Autodesk Fusion 360 part; units mm, degrees
note: some values were not read from the file. Set by a fixed rule: which sketch regions a step uses.
(part 2 of 3)
  line L685 (14.5126, 3.5841) -> (14.4849, 3.5912)
  line L686 (14.4849, 0.409) -> (14.5126, 0.4161)
  line L687 (11.4493, 3.5709) -> (11.4223, 3.5588)
  line L688 (11.209, 0.715) -> (11.2161, 0.6873)
  line L689 (11.5713, 0.4011) -> (11.5999, 0.4001)
  line L690 (14.4568, 0.4039) -> (14.4849, 0.409)
  line L691 (11.3477, 3.5108) -> (11.3254, 3.4913)
  line L692 (14.7988, 0.7713) -> (14.7998, 0.7998)
  line L693 (14.7509, 0.6082) -> (14.7637, 0.6337)
  line L694 (11.2097, 3.2885) -> (11.2043, 3.2594)
  line L695 (14.7022, 0.5379) -> (14.7201, 0.5601)
  line L696 (14.6618, 0.4976) -> (14.6827, 0.517)
  line L697 (14.6827, 0.517) -> (14.7022, 0.5379)
  line L698 (14.5126, 0.4161) -> (14.5397, 0.4251)
  line L699 (14.5916, 0.4488) -> (14.6161, 0.4634)
  line L700 (14.5397, 0.4251) -> (14.566, 0.436)
  line L701 (14.6161, 0.4634) -> (14.6396, 0.4796)
  line L702 (14.7998, 0.7998) -> (14.7998, 3.2004)
  line L703 (14.7836, 0.6872) -> (14.7907, 0.7148)
  line L704 (34.6396, 3.5206) -> (34.6161, 3.5368)
  line L705 (31.4337, 0.4362) -> (31.4601, 0.4253)
  line L706 (31.2634, 0.5838) -> (31.2797, 0.5603)
  line L707 (34.7201, 0.5601) -> (34.7364, 0.5836)
  line L708 (31.4771, 3.581) -> (31.4493, 3.5709)
  line L709 (31.4601, 0.4253) -> (31.4872, 0.4163)
  line L710 (34.3999, 0.3998) -> (34.4284, 0.4009)
  line L711 (31.1999, 3.2001) -> (31.1999, 0.8)
  line L712 (34.6396, 0.4796) -> (34.6618, 0.4976)
  line L713 (31.317, 0.5172) -> (31.3379, 0.4977)
  line L714 (34.7364, 0.5836) -> (34.7509, 0.6082)
  line L715 (31.4082, 0.449) -> (31.4337, 0.4362)
  line L716 (31.564, 3.5987) -> (31.5346, 3.595)
  line L717 (34.6618, 3.5026) -> (34.6396, 3.5206)
  line L718 (34.4284, 3.5993) -> (34.3999, 3.6004)
  line L719 (31.3962, 3.5446) -> (31.3713, 3.5286)
  line L720 (31.3379, 0.4977) -> (31.3602, 0.4798)
  line L721 (34.4284, 0.4009) -> (34.4568, 0.4039)
  line L722 (34.7988, 0.7713) -> (34.7998, 0.7998)
  line L723 (34.5126, 0.4161) -> (34.5397, 0.4251)
  line L724 (31.2097, 3.2885) -> (31.2043, 3.2594)
  line L725 (31.2161, 0.6873) -> (31.2251, 0.6602)
  line L726 (34.4568, 0.4039) -> (34.4849, 0.409)
  line L727 (31.2488, 0.6083) -> (31.2634, 0.5838)
  line L728 (31.1999, 3.2005) -> (31.1999, 3.2001)
  line L729 (31.3836, 0.4635) -> (31.4082, 0.449)
  line L730 (34.4849, 0.409) -> (34.5126, 0.4161)
  line L731 (34.6827, 0.517) -> (34.7022, 0.5379)
  line L732 (31.2009, 0.7715) -> (31.2039, 0.7431)
  line L733 (31.2797, 0.5603) -> (31.2976, 0.5381)
  line L734 (31.209, 0.715) -> (31.2161, 0.6873)
  line L735 (31.2976, 0.5381) -> (31.317, 0.5172)
  line L736 (31.1999, 3.2004) -> (31.1999, 3.2005)
  line L737 (34.3999, 0.4001) -> (34.3999, 0.3998)
  line L738 (34.7637, 0.6337) -> (34.7746, 0.6601)
  line L739 (34.7907, 0.7148) -> (34.7958, 0.7429)
  line L740 (34.7958, 0.7429) -> (34.7988, 0.7713)
  line L741 (34.5916, 0.4488) -> (34.6161, 0.4634)
  line L742 (34.7836, 0.6872) -> (34.7907, 0.7148)
  line L743 (34.5397, 0.4251) -> (34.566, 0.436)
  line L744 (34.6618, 0.4976) -> (34.6827, 0.517)
  line L745 (34.7998, 0.7998) -> (34.7998, 3.2004)
  line L746 (34.7958, 3.2573) -> (34.7907, 3.2854)
  line L747 (34.7836, 3.313) -> (34.7746, 3.3401)
  line L748 (34.6161, 3.5368) -> (34.5916, 3.5514)
  line L749 (31.5346, 3.595) -> (31.5056, 3.5891)
  line L750 (34.3999, 3.6004) -> (34.3999, 3.6002)
  line L751 (31.3046, 3.4702) -> (31.2855, 3.4476)
  line L752 (31.268, 3.4237) -> (31.2524, 3.3985)
  line L753 (34.7201, 3.4401) -> (34.7022, 3.4623)
  line L754 (31.2524, 3.3985) -> (31.2387, 3.3723)
  line L755 (34.7998, 3.2004) -> (34.7988, 3.2289)
  line L756 (31.227, 3.3451) -> (31.2173, 3.3171)
  line L757 (34.5916, 3.5514) -> (34.566, 3.5642)
  line L758 (31.3713, 3.5286) -> (31.3477, 3.5108)
  line L759 (31.4493, 3.5709) -> (31.4223, 3.5588)
  line L760 (34.7988, 3.2289) -> (34.7958, 3.2573)
  line L761 (34.3999, 3.6002) -> (31.5999, 3.6002)
  line L762 (31.4223, 3.5588) -> (31.3962, 3.5446)
  line L763 (34.7637, 3.3665) -> (34.7509, 3.392)
  line L764 (34.7022, 3.4623) -> (34.6827, 3.4832)
  line L765 (31.3254, 3.4913) -> (31.3046, 3.4702)
  line L766 (34.7364, 3.4166) -> (34.7201, 3.4401)
  line L767 (34.7509, 3.392) -> (34.7364, 3.4166)
  line L768 (34.7746, 3.3401) -> (34.7637, 3.3665)
  line L769 (31.5935, 3.6003) -> (31.564, 3.5987)
  line L770 (31.3477, 3.5108) -> (31.3254, 3.4913)
  line L771 (31.2173, 3.3171) -> (31.2097, 3.2885)
  line L772 (34.5126, 3.5841) -> (34.4849, 3.5912)
  line L773 (31.5999, 3.6002) -> (31.5935, 3.6003)
  line L774 (31.5056, 3.5891) -> (31.4771, 3.581)
  line L775 (31.4872, 0.4163) -> (31.5149, 0.4092)
  line L776 (31.2387, 3.3723) -> (31.227, 3.3451)
  line L777 (31.201, 3.2299) -> (31.1999, 3.2004)
  line L778 (34.7907, 3.2854) -> (34.7836, 3.313)
  line L779 (31.1999, 0.8) -> (31.2009, 0.7715)
  line L780 (34.5397, 3.5751) -> (34.5126, 3.5841)
  line L781 (34.566, 3.5642) -> (34.5397, 3.5751)
  line L782 (34.6161, 0.4634) -> (34.6396, 0.4796)
  line L783 (34.6827, 3.4832) -> (34.6618, 3.5026)
  line L784 (31.3602, 0.4798) -> (31.3836, 0.4635)
  line L785 (34.4849, 3.5912) -> (34.4568, 3.5963)
  line L786 (34.4568, 3.5963) -> (34.4284, 3.5993)
  line L787 (31.2855, 3.4476) -> (31.268, 3.4237)
  line L788 (34.566, 0.436) -> (34.5916, 0.4488)
  line L789 (34.7746, 0.6601) -> (34.7836, 0.6872)
  line L790 (31.2039, 0.7431) -> (31.209, 0.715)
  line L791 (31.2043, 3.2594) -> (31.201, 3.2299)
  line L792 (31.2251, 0.6602) -> (31.236, 0.6339)
  line L793 (31.5999, 0.4001) -> (34.3999, 0.4001)
  line L794 (31.5713, 0.4011) -> (31.5999, 0.4001)
  line L795 (31.236, 0.6339) -> (31.2488, 0.6083)
  line L796 (31.5149, 0.4092) -> (31.5429, 0.4041)
  line L797 (34.7022, 0.5379) -> (34.7201, 0.5601)
  line L798 (34.7509, 0.6082) -> (34.7637, 0.6337)
  line L799 (31.5429, 0.4041) -> (31.5713, 0.4011)
  line L800 (51.4223, 3.5588) -> (51.3962, 3.5446)
  line L801 (54.7201, 3.4401) -> (54.7022, 3.4623)
  line L802 (51.3254, 3.4913) -> (51.3046, 3.4702)
  line L803 (51.2855, 3.4476) -> (51.268, 3.4237)
  line L804 (51.2524, 3.3985) -> (51.2387, 3.3723)
  line L805 (54.7637, 0.6337) -> (54.7746, 0.6601)
  line L806 (54.566, 3.5642) -> (54.5397, 3.5751)
  line L807 (51.2797, 0.5603) -> (51.2976, 0.5381)
  line L808 (54.7988, 0.7713) -> (54.7998, 0.7998)
  line L809 (51.317, 0.5172) -> (51.3379, 0.4977)
  line L810 (54.3999, 3.6004) -> (54.3999, 3.6002)
  line L811 (51.3602, 0.4798) -> (51.3836, 0.4635)
  line L812 (54.6161, 0.4634) -> (54.6396, 0.4796)
  line L813 (54.7907, 0.7148) -> (54.7958, 0.7429)
  line L814 (54.7998, 0.7998) -> (54.7998, 3.2004)
  line L815 (54.7022, 3.4623) -> (54.6827, 3.4832)
  line L816 (51.2039, 0.7431) -> (51.209, 0.715)
  line L817 (54.7988, 3.2289) -> (54.7958, 3.2573)
  line L818 (51.5346, 3.595) -> (51.5056, 3.5891)
  line L819 (51.227, 3.3451) -> (51.2173, 3.3171)
  line L820 (54.7022, 0.5379) -> (54.7201, 0.5601)
  line L821 (54.6618, 0.4976) -> (54.6827, 0.517)
  line L822 (54.6396, 3.5206) -> (54.6161, 3.5368)
  line L823 (54.4284, 0.4009) -> (54.4568, 0.4039)
  line L824 (54.7201, 0.5601) -> (54.7364, 0.5836)
  line L825 (54.7509, 0.6082) -> (54.7637, 0.6337)
  line L826 (54.4568, 0.4039) -> (54.4849, 0.409)
  line L827 (51.5999, 0.4001) -> (54.3999, 0.4001)
  line L828 (54.7958, 0.7429) -> (54.7988, 0.7713)
  line L829 (54.5916, 0.4488) -> (54.6161, 0.4634)
  line L830 (51.4601, 0.4253) -> (51.4872, 0.4163)
  line L831 (54.6618, 3.5026) -> (54.6396, 3.5206)
  line L832 (54.5126, 3.5841) -> (54.4849, 3.5912)
  line L833 (51.3713, 3.5286) -> (51.3477, 3.5108)
  line L834 (54.4849, 0.409) -> (54.5126, 0.4161)
  line L835 (54.5916, 3.5514) -> (54.566, 3.5642)
  line L836 (54.3999, 3.6002) -> (51.5999, 3.6002)
  line L837 (51.4493, 3.5709) -> (51.4223, 3.5588)
  line L838 (54.7836, 0.6872) -> (54.7907, 0.7148)
  line L839 (54.7364, 0.5836) -> (54.7509, 0.6082)
  line L840 (51.2097, 3.2885) -> (51.2043, 3.2594)
  line L841 (51.2043, 3.2594) -> (51.201, 3.2299)
  line L842 (54.4284, 3.5993) -> (54.3999, 3.6004)
  line L843 (51.3379, 0.4977) -> (51.3602, 0.4798)
  line L844 (51.5149, 0.4092) -> (51.5429, 0.4041)
  line L845 (51.4082, 0.449) -> (51.4337, 0.4362)
  line L846 (51.3836, 0.4635) -> (51.4082, 0.449)
  line L847 (51.564, 3.5987) -> (51.5346, 3.595)
  line L848 (54.4568, 3.5963) -> (54.4284, 3.5993)
  line L849 (51.5429, 0.4041) -> (51.5713, 0.4011)
  line L850 (51.236, 0.6339) -> (51.2488, 0.6083)
  line L851 (54.7907, 3.2854) -> (54.7836, 3.313)
  line L852 (51.4337, 0.4362) -> (51.4601, 0.4253)
  line L853 (54.7746, 3.3401) -> (54.7637, 3.3665)
  line L854 (51.2387, 3.3723) -> (51.227, 3.3451)
  line L855 (54.7637, 3.3665) -> (54.7509, 3.392)
  line L856 (51.4771, 3.581) -> (51.4493, 3.5709)
  line L857 (54.7958, 3.2573) -> (54.7907, 3.2854)
  line L858 (54.7998, 3.2004) -> (54.7988, 3.2289)
  line L859 (51.2173, 3.3171) -> (51.2097, 3.2885)
  line L860 (51.5999, 3.6002) -> (51.5935, 3.6003)
  line L861 (51.2634, 0.5838) -> (51.2797, 0.5603)
  line L862 (51.5713, 0.4011) -> (51.5999, 0.4001)
  line L863 (54.6161, 3.5368) -> (54.5916, 3.5514)
  line L864 (51.1999, 3.2005) -> (51.1999, 3.2001)
  line L865 (51.201, 3.2299) -> (51.1999, 3.2004)
  line L866 (54.6827, 3.4832) -> (54.6618, 3.5026)
  line L867 (51.2009, 0.7715) -> (51.2039, 0.7431)
  line L868 (51.268, 3.4237) -> (51.2524, 3.3985)
  line L869 (51.3477, 3.5108) -> (51.3254, 3.4913)
  line L870 (54.7836, 3.313) -> (54.7746, 3.3401)
  line L871 (54.7364, 3.4166) -> (54.7201, 3.4401)
  line L872 (54.7509, 3.392) -> (54.7364, 3.4166)
  line L873 (51.3046, 3.4702) -> (51.2855, 3.4476)
  line L874 (51.1999, 0.8) -> (51.2009, 0.7715)
  line L875 (51.1999, 3.2001) -> (51.1999, 0.8)
  line L876 (51.5056, 3.5891) -> (51.4771, 3.581)
  line L877 (51.2488, 0.6083) -> (51.2634, 0.5838)
  line L878 (51.2976, 0.5381) -> (51.317, 0.5172)
  line L879 (54.566, 0.436) -> (54.5916, 0.4488)
  line L880 (51.5935, 3.6003) -> (51.564, 3.5987)
  line L881 (51.209, 0.715) -> (51.2161, 0.6873)
  line L882 (51.1999, 3.2004) -> (51.1999, 3.2005)
  line L883 (54.6827, 0.517) -> (54.7022, 0.5379)
  line L884 (54.7746, 0.6601) -> (54.7836, 0.6872)
  line L885 (54.3999, 0.3998) -> (54.4284, 0.4009)
  line L886 (54.5397, 0.4251) -> (54.566, 0.436)
  line L887 (51.3962, 3.5446) -> (51.3713, 3.5286)
  line L888 (54.6396, 0.4796) -> (54.6618, 0.4976)
  line L889 (54.4849, 3.5912) -> (54.4568, 3.5963)
  line L890 (54.5126, 0.4161) -> (54.5397, 0.4251)
  line L891 (51.2161, 0.6873) -> (51.2251, 0.6602)
  line L892 (51.4872, 0.4163) -> (51.5149, 0.4092)
  line L893 (54.3999, 0.4001) -> (54.3999, 0.3998)
  line L894 (54.5397, 3.5751) -> (54.5126, 3.5841)
  line L895 (51.2251, 0.6602) -> (51.236, 0.6339)
  line L896 (74.7637, 3.3665) -> (74.7509, 3.392)
  line L897 (74.7958, 3.2573) -> (74.7907, 3.2854)
  line L898 (71.3962, 3.5446) -> (71.3713, 3.5286)
  line L899 (71.5056, 3.5891) -> (71.4771, 3.581)
  line L900 (71.564, 3.5987) -> (71.5346, 3.595)
  line L901 (71.4223, 3.5588) -> (71.3962, 3.5446)
  line L902 (74.4568, 3.5963) -> (74.4284, 3.5993)
  line L903 (74.7509, 3.392) -> (74.7364, 3.4166)
  line L904 (71.4493, 3.5709) -> (71.4223, 3.5588)
  line L905 (71.5346, 3.595) -> (71.5056, 3.5891)
  line L906 (74.6618, 3.5026) -> (74.6396, 3.5206)
  line L907 (71.5429, 0.4041) -> (71.5713, 0.4011)
  line L908 (74.5916, 0.4488) -> (74.6161, 0.4634)
  line L909 (74.3999, 3.6004) -> (74.3999, 3.6002)
  line L910 (74.6396, 3.5206) -> (74.6161, 3.5368)
  line L911 (74.6827, 3.4832) -> (74.6618, 3.5026)
  line L912 (74.7836, 0.6872) -> (74.7907, 0.7148)
  line L913 (71.3602, 0.4798) -> (71.3836, 0.4635)
  line L914 (71.209, 0.715) -> (71.2161, 0.6873)
  line L915 (71.2251, 0.6602) -> (71.236, 0.6339)
  line L916 (71.4872, 0.4163) -> (71.5149, 0.4092)
  line L917 (71.5149, 0.4092) -> (71.5429, 0.4041)
  line L918 (74.6618, 0.4976) -> (74.6827, 0.517)
  line L919 (74.7364, 0.5836) -> (74.7509, 0.6082)
  line L920 (74.7958, 0.7429) -> (74.7988, 0.7713)
  line L921 (71.4771, 3.581) -> (71.4493, 3.5709)
  line L922 (71.236, 0.6339) -> (71.2488, 0.6083)
  line L923 (74.3999, 0.4001) -> (74.3999, 0.3998)
  line L924 (71.3713, 3.5286) -> (71.3477, 3.5108)
  line L925 (74.5916, 3.5514) -> (74.566, 3.5642)
  line L926 (74.7022, 3.4623) -> (74.6827, 3.4832)
  line L927 (74.566, 3.5642) -> (74.5397, 3.5751)
  line L928 (71.2488, 0.6083) -> (71.2634, 0.5838)
  line L929 (71.2797, 0.5603) -> (71.2976, 0.5381)
  line L930 (74.6161, 0.4634) -> (74.6396, 0.4796)
  line L931 (74.4849, 3.5912) -> (74.4568, 3.5963)
  line L932 (74.7988, 0.7713) -> (74.7998, 0.7998)
  line L933 (74.6827, 0.517) -> (74.7022, 0.5379)
  line L934 (74.566, 0.436) -> (74.5916, 0.4488)
  line L935 (71.5999, 0.4001) -> (74.3999, 0.4001)
  line L936 (74.4568, 0.4039) -> (74.4849, 0.409)
  line L937 (71.2009, 0.7715) -> (71.2039, 0.7431)
  line L938 (71.2387, 3.3723) -> (71.227, 3.3451)
  line L939 (74.7201, 0.5601) -> (74.7364, 0.5836)
  line L940 (71.201, 3.2299) -> (71.1999, 3.2004)
  line L941 (74.7022, 0.5379) -> (74.7201, 0.5601)
  line L942 (74.4849, 0.409) -> (74.5126, 0.4161)
  line L943 (71.3379, 0.4977) -> (71.3602, 0.4798)
  line L944 (71.268, 3.4237) -> (71.2524, 3.3985)
  line L945 (71.3836, 0.4635) -> (71.4082, 0.449)
  line L946 (71.4601, 0.4253) -> (71.4872, 0.4163)
  line L947 (74.7746, 0.6601) -> (74.7836, 0.6872)
  line L948 (71.5713, 0.4011) -> (71.5999, 0.4001)
  line L949 (74.7907, 3.2854) -> (74.7836, 3.313)
  line L950 (71.2173, 3.3171) -> (71.2097, 3.2885)
  line L951 (71.2043, 3.2594) -> (71.201, 3.2299)
  line L952 (74.7907, 0.7148) -> (74.7958, 0.7429)
  line L953 (74.6161, 3.5368) -> (74.5916, 3.5514)
  line L954 (74.7637, 0.6337) -> (74.7746, 0.6601)
  line L955 (74.7509, 0.6082) -> (74.7637, 0.6337)
  line L956 (71.2524, 3.3985) -> (71.2387, 3.3723)
  line L957 (71.4337, 0.4362) -> (71.4601, 0.4253)
  line L958 (71.227, 3.3451) -> (71.2173, 3.3171)
  line L959 (71.1999, 3.2004) -> (71.1999, 3.2005)
  line L960 (74.5397, 0.4251) -> (74.566, 0.436)
  line L961 (74.5126, 0.4161) -> (74.5397, 0.4251)
  line L962 (71.2161, 0.6873) -> (71.2251, 0.6602)
  line L963 (71.2634, 0.5838) -> (71.2797, 0.5603)
  line L964 (71.1999, 0.8) -> (71.2009, 0.7715)
  line L965 (71.1999, 3.2001) -> (71.1999, 0.8)
  line L966 (71.2039, 0.7431) -> (71.209, 0.715)
  line L967 (74.4284, 0.4009) -> (74.4568, 0.4039)
  line L968 (71.317, 0.5172) -> (71.3379, 0.4977)
  line L969 (74.7998, 0.7998) -> (74.7998, 3.2004)
  line L970 (74.6396, 0.4796) -> (74.6618, 0.4976)
  line L971 (71.2976, 0.5381) -> (71.317, 0.5172)
  line L972 (71.4082, 0.449) -> (71.4337, 0.4362)
  line L973 (71.1999, 3.2005) -> (71.1999, 3.2001)
  line L974 (74.3999, 0.3998) -> (74.4284, 0.4009)
  line L975 (71.2097, 3.2885) -> (71.2043, 3.2594)
  line L976 (74.3999, 3.6002) -> (71.5999, 3.6002)
  line L977 (74.7364, 3.4166) -> (74.7201, 3.4401)
  line L978 (71.3254, 3.4913) -> (71.3046, 3.4702)
  line L979 (74.7746, 3.3401) -> (74.7637, 3.3665)
  line L980 (74.7836, 3.313) -> (74.7746, 3.3401)
  line L981 (71.3046, 3.4702) -> (71.2855, 3.4476)
  line L982 (74.5126, 3.5841) -> (74.4849, 3.5912)
  line L983 (74.7988, 3.2289) -> (74.7958, 3.2573)
  line L984 (71.5999, 3.6002) -> (71.5935, 3.6003)
  line L985 (74.5397, 3.5751) -> (74.5126, 3.5841)
  line L986 (71.3477, 3.5108) -> (71.3254, 3.4913)
  line L987 (71.5935, 3.6003) -> (71.564, 3.5987)
  line L988 (74.4284, 3.5993) -> (74.3999, 3.6004)
  line L989 (71.2855, 3.4476) -> (71.268, 3.4237)
  line L990 (74.7201, 3.4401) -> (74.7022, 3.4623)
  line L991 (74.7998, 3.2004) -> (74.7988, 3.2289)
  line L992 (83.2001, 14.4001) -> (83.2001, 11.6001)
  line L993 (83.236, 11.434) -> (83.2488, 11.4084)
  line L994 (83.2488, 11.4084) -> (83.2634, 11.3839)
  line L995 (83.2041, 14.4571) -> (83.2011, 14.4287)
  line L996 (86.3891, 14.4944) -> (86.381, 14.5229)
  line L997 (86.3751, 11.4603) -> (86.3841, 11.4874)
  line L998 (83.2976, 11.3382) -> (83.317, 11.3173)
  line L999 (86.3963, 11.5432) -> (86.3993, 11.5716)
  line L1000 (83.5148, 11.2093) -> (83.5429, 11.2042)
  line L1001 (86.1401, 11.2254) -> (86.1665, 11.2363)
  line L1002 (86.2913, 14.6746) -> (86.2702, 14.6954)
  line L1003 (86.1985, 14.7476) -> (86.1723, 14.7613)
  line L1004 (86.3368, 11.3839) -> (86.3514, 11.4084)
  line L1005 (86.0299, 14.799) -> (86.0004, 14.8001)
  line L1006 (86.0594, 14.7957) -> (86.0299, 14.799)
  line L1007 (83.2161, 11.4874) -> (83.2251, 11.4603)
  line L1008 (86.1723, 14.7613) -> (86.1451, 14.773)
  line L1009 (83.249, 14.5918) -> (83.2362, 14.5663)
  line L1010 (86.3588, 14.5777) -> (86.3446, 14.6038)
  line L1011 (83.209, 11.5151) -> (83.2161, 11.4874)
  line L1012 (83.2634, 11.3839) -> (83.2796, 11.3604)
  line L1013 (83.317, 11.3173) -> (83.3379, 11.2978)
  line L1014 (83.4601, 11.2254) -> (83.4872, 11.2164)
  line L1015 (83.3601, 11.2799) -> (83.3836, 11.2636)
  line L1016 (83.4337, 11.2363) -> (83.4601, 11.2254)
  line L1017 (86.4004, 11.6001) -> (86.4002, 11.6001)
  line L1018 (86.2401, 11.2799) -> (86.2623, 11.2978)
  line L1019 (86.1451, 14.773) -> (86.1171, 14.7827)
  line L1020 (83.2092, 14.4851) -> (83.2041, 14.4571)
  line L1021 (83.2251, 11.4603) -> (83.236, 11.434)
  line L1022 (86.0885, 14.7903) -> (86.0594, 14.7957)
  line L1023 (86.0573, 11.2042) -> (86.0854, 11.2093)
  line L1024 (83.2977, 14.6621) -> (83.2798, 14.6398)
  line L1025 (86.0005, 14.8001) -> (86.0001, 14.8001)
  line L1026 (83.2796, 11.3604) -> (83.2976, 11.3382)
  line L1027 (83.2039, 11.5432) -> (83.209, 11.5151)
  line L1028 (86.0004, 14.8001) -> (86.0005, 14.8001)
  line L1029 (86.3446, 14.6038) -> (86.3286, 14.6287)
  line L1030 (83.5998, 11.2002) -> (86.0004, 11.2002)
  line L1031 (86.2832, 11.3173) -> (86.3026, 11.3382)
  line L1032 (86.1171, 14.7827) -> (86.0885, 14.7903)
  line L1033 (86.4003, 14.4065) -> (86.3987, 14.436)
  line L1034 (86.395, 14.4654) -> (86.3891, 14.4944)
  line L1035 (86.3206, 11.3604) -> (86.3368, 11.3839)
  line L1036 (86.3993, 11.5716) -> (86.4004, 11.6001)
  line L1037 (83.5431, 14.7961) -> (83.515, 14.791)
  line L1038 (83.4082, 11.2491) -> (83.4337, 11.2363)
  line L1039 (86.3709, 14.5507) -> (86.3588, 14.5777)
  line L1040 (83.4873, 14.7839) -> (83.4602, 14.7749)
  line L1041 (86.4002, 14.4001) -> (86.4003, 14.4065)
  line L1042 (83.4602, 14.7749) -> (83.4339, 14.764)
  line L1043 (83.2001, 11.6001) -> (83.1998, 11.6001)
  line L1044 (83.2011, 14.4287) -> (83.2001, 14.4001)
  line L1045 (86.3987, 14.436) -> (86.395, 14.4654)
  line L1046 (86.2237, 14.732) -> (86.1985, 14.7476)
  line L1047 (83.3172, 14.683) -> (83.2977, 14.6621)
  line L1048 (86.2476, 14.7145) -> (86.2237, 14.732)
  line L1049 (83.515, 14.791) -> (83.4873, 14.7839)
  line L1050 (86.2702, 14.6954) -> (86.2476, 14.7145)
  line L1051 (83.2635, 14.6164) -> (83.249, 14.5918)
  line L1052 (83.5715, 14.7991) -> (83.5431, 14.7961)
  line L1053 (83.3838, 14.7366) -> (83.3603, 14.7203)
  line L1054 (83.5429, 11.2042) -> (83.5713, 11.2012)
  line L1055 (83.2798, 14.6398) -> (83.2635, 14.6164)
  line L1056 (83.2163, 14.5128) -> (83.2092, 14.4851)
  line L1057 (83.5713, 11.2012) -> (83.5998, 11.2002)
  line L1058 (86.3841, 11.4874) -> (86.3912, 11.5151)
  line L1059 (83.6, 14.8001) -> (83.5715, 14.7991)
  line L1060 (83.4083, 14.7512) -> (83.3838, 14.7366)
  line L1061 (83.3381, 14.7024) -> (83.3172, 14.683)
  line L1062 (83.2009, 11.5716) -> (83.2039, 11.5432)
  line L1063 (83.4339, 14.764) -> (83.4083, 14.7512)
  line L1064 (86.3912, 11.5151) -> (86.3963, 11.5432)
  line L1065 (86.3642, 11.434) -> (86.3751, 11.4603)
  line L1066 (83.1998, 11.6001) -> (83.2009, 11.5716)
  line L1067 (83.2253, 14.5399) -> (83.2163, 14.5128)
  line L1068 (86.192, 11.2491) -> (86.2166, 11.2636)
  line L1069 (83.3379, 11.2978) -> (83.3601, 11.2799)
  line L1070 (86.4002, 11.6001) -> (86.4002, 14.4001)
  line L1071 (86.381, 14.5229) -> (86.3709, 14.5507)
  line L1072 (86.3026, 11.3382) -> (86.3206, 11.3604)
  line L1073 (83.3836, 11.2636) -> (83.4082, 11.2491)
  line L1074 (83.2362, 14.5663) -> (83.2253, 14.5399)
  line L1075 (83.4872, 11.2164) -> (83.5148, 11.2093)
  line L1076 (86.0004, 11.2002) -> (86.0289, 11.2012)
  line L1077 (86.2166, 11.2636) -> (86.2401, 11.2799)
  line L1078 (86.3108, 14.6523) -> (86.2913, 14.6746)
  line L1079 (86.0854, 11.2093) -> (86.113, 11.2164)
  line L1080 (83.3603, 14.7203) -> (83.3381, 14.7024)
  line L1081 (86.2623, 11.2978) -> (86.2832, 11.3173)
  line L1082 (86.3514, 11.4084) -> (86.3642, 11.434)
  line L1083 (86.3286, 14.6287) -> (86.3108, 14.6523)
  line L1084 (86.0001, 14.8001) -> (83.6, 14.8001)
  line L1085 (86.0289, 11.2012) -> (86.0573, 11.2042)
  line L1086 (86.113, 11.2164) -> (86.1401, 11.2254)
  line L1087 (86.1665, 11.2363) -> (86.192, 11.2491)
  line L1088 (86.4004, 31.6001) -> (86.4002, 31.6001)
  line L1089 (86.4002, 31.6001) -> (86.4002, 34.4001)
  line L1090 (86.2166, 31.2636) -> (86.2401, 31.2799)
  line L1091 (86.3206, 31.3604) -> (86.3368, 31.3839)
  line L1092 (86.192, 31.2491) -> (86.2166, 31.2636)
  line L1093 (83.2977, 34.6621) -> (83.2798, 34.6398)
  line L1094 (83.2798, 34.6398) -> (83.2635, 34.6164)
  line L1095 (86.4003, 34.4065) -> (86.3987, 34.436)
  line L1096 (86.3751, 31.4603) -> (86.3841, 31.4874)
  line L1097 (86.0854, 31.2093) -> (86.113, 31.2164)
  line L1098 (86.0004, 31.2002) -> (86.0289, 31.2012)
  line L1099 (83.2796, 31.3604) -> (83.2976, 31.3382)
  line L1100 (83.4082, 31.2491) -> (83.4337, 31.2363)
  line L1101 (86.381, 34.5229) -> (86.3709, 34.5507)
  line L1102 (83.2011, 34.4287) -> (83.2001, 34.4001)
  line L1103 (86.3987, 34.436) -> (86.395, 34.4654)
  line L1104 (86.395, 34.4654) -> (86.3891, 34.4944)
  line L1105 (83.2009, 31.5716) -> (83.2039, 31.5432)
  line L1106 (86.3912, 31.5151) -> (86.3963, 31.5432)
  line L1107 (86.1401, 31.2254) -> (86.1665, 31.2363)
  line L1108 (86.3368, 31.3839) -> (86.3514, 31.4084)
  line L1109 (83.2001, 31.6001) -> (83.1998, 31.6001)
  line L1110 (86.2832, 31.3173) -> (86.3026, 31.3382)
  line L1111 (86.0573, 31.2042) -> (86.0854, 31.2093)
  line L1112 (86.113, 31.2164) -> (86.1401, 31.2254)
  line L1113 (83.4601, 31.2254) -> (83.4872, 31.2164)
  line L1114 (83.2161, 31.4874) -> (83.2251, 31.4603)
  line L1115 (83.2976, 31.3382) -> (83.317, 31.3173)
  line L1116 (83.3379, 31.2978) -> (83.3601, 31.2799)
  line L1117 (86.0005, 34.8001) -> (86.0001, 34.8001)
  line L1118 (83.1998, 31.6001) -> (83.2009, 31.5716)
  line L1119 (83.4083, 34.7512) -> (83.3838, 34.7366)
  line L1120 (83.4872, 31.2164) -> (83.5148, 31.2093)
  line L1121 (86.2237, 34.732) -> (86.1985, 34.7476)
  line L1122 (86.3709, 34.5507) -> (86.3588, 34.5777)
  line L1123 (86.3963, 31.5432) -> (86.3993, 31.5716)
  line L1124 (83.2634, 31.3839) -> (83.2796, 31.3604)
  line L1125 (86.0289, 31.2012) -> (86.0573, 31.2042)
  line L1126 (86.3588, 34.5777) -> (86.3446, 34.6038)
  line L1127 (86.1451, 34.773) -> (86.1171, 34.7827)
  line L1128 (86.4002, 34.4001) -> (86.4003, 34.4065)
  line L1129 (83.515, 34.791) -> (83.4873, 34.7839)
  line L1130 (83.4339, 34.764) -> (83.4083, 34.7512)
  line L1131 (83.5148, 31.2093) -> (83.5429, 31.2042)
  line L1132 (83.2253, 34.5399) -> (83.2163, 34.5128)
  line L1133 (86.3026, 31.3382) -> (86.3206, 31.3604)
  line L1134 (86.3514, 31.4084) -> (86.3642, 31.434)
  line L1135 (83.5431, 34.7961) -> (83.515, 34.791)
  line L1136 (86.3841, 31.4874) -> (86.3912, 31.5151)
  line L1137 (86.3993, 31.5716) -> (86.4004, 31.6001)
  line L1138 (86.3642, 31.434) -> (86.3751, 31.4603)
  line L1139 (83.2635, 34.6164) -> (83.249, 34.5918)
  line L1140 (86.1171, 34.7827) -> (86.0885, 34.7903)
  line L1141 (86.1723, 34.7613) -> (86.1451, 34.773)
  line L1142 (83.209, 31.5151) -> (83.2161, 31.4874)
  line L1143 (86.0299, 34.799) -> (86.0004, 34.8001)
  line L1144 (83.6, 34.8001) -> (83.5715, 34.7991)
  line L1145 (86.2913, 34.6746) -> (86.2702, 34.6954)
  line L1146 (83.2039, 31.5432) -> (83.209, 31.5151)
  line L1147 (83.317, 31.3173) -> (83.3379, 31.2978)
  line L1148 (86.3108, 34.6523) -> (86.2913, 34.6746)
  line L1149 (83.2362, 34.5663) -> (83.2253, 34.5399)
  line L1150 (83.2251, 31.4603) -> (83.236, 31.434)
  line L1151 (83.236, 31.434) -> (83.2488, 31.4084)
  line L1152 (86.0004, 34.8001) -> (86.0005, 34.8001)
  line L1153 (83.4337, 31.2363) -> (83.4601, 31.2254)
  line L1154 (83.2488, 31.4084) -> (83.2634, 31.3839)
  line L1155 (83.3603, 34.7203) -> (83.3381, 34.7024)
  line L1156 (83.3836, 31.2636) -> (83.4082, 31.2491)
  line L1157 (83.2041, 34.4571) -> (83.2011, 34.4287)
  line L1158 (86.0594, 34.7957) -> (86.0299, 34.799)
  line L1159 (83.5713, 31.2012) -> (83.5998, 31.2002)
  line L1160 (86.3286, 34.6287) -> (86.3108, 34.6523)
  line L1161 (86.3891, 34.4944) -> (86.381, 34.5229)
  line L1162 (83.5429, 31.2042) -> (83.5713, 31.2012)
  line L1163 (83.249, 34.5918) -> (83.2362, 34.5663)
  line L1164 (83.2001, 34.4001) -> (83.2001, 31.6001)
  line L1165 (83.2092, 34.4851) -> (83.2041, 34.4571)
  line L1166 (86.1985, 34.7476) -> (86.1723, 34.7613)
  line L1167 (86.2476, 34.7145) -> (86.2237, 34.732)
  line L1168 (83.5998, 31.2002) -> (86.0004, 31.2002)
  line L1169 (86.0001, 34.8001) -> (83.6, 34.8001)
  line L1170 (83.2163, 34.5128) -> (83.2092, 34.4851)
  line L1171 (86.0885, 34.7903) -> (86.0594, 34.7957)
  line L1172 (83.3381, 34.7024) -> (83.3172, 34.683)
  line L1173 (83.5715, 34.7991) -> (83.5431, 34.7961)
  line L1174 (86.3446, 34.6038) -> (86.3286, 34.6287)
  line L1175 (83.3601, 31.2799) -> (83.3836, 31.2636)
  line L1176 (86.2623, 31.2978) -> (86.2832, 31.3173)
  line L1177 (86.1665, 31.2363) -> (86.192, 31.2491)
  line L1178 (86.2401, 31.2799) -> (86.2623, 31.2978)
  line L1179 (83.3172, 34.683) -> (83.2977, 34.6621)
  line L1180 (83.4873, 34.7839) -> (83.4602, 34.7749)
  line L1181 (83.3838, 34.7366) -> (83.3603, 34.7203)
  line L1182 (86.2702, 34.6954) -> (86.2476, 34.7145)
  line L1183 (83.4602, 34.7749) -> (83.4339, 34.764)
  line L1184 (83.249, 54.5918) -> (83.2362, 54.5663)
  line L1185 (86.2913, 54.6746) -> (86.2702, 54.6954)
  line L1186 (83.3601, 51.2799) -> (83.3836, 51.2636)
  line L1187 (83.3836, 51.2636) -> (83.4082, 51.2491)
  line L1188 (83.5713, 51.2012) -> (83.5998, 51.2002)
  line L1189 (83.4601, 51.2254) -> (83.4872, 51.2164)
  line L1190 (86.3108, 54.6523) -> (86.2913, 54.6746)
  line L1191 (86.1985, 54.7476) -> (86.1723, 54.7613)
  line L1192 (83.5998, 51.2002) -> (86.0004, 51.2002)
  line L1193 (86.0004, 51.2002) -> (86.0289, 51.2012)
  line L1194 (86.113, 51.2164) -> (86.1401, 51.2254)
  line L1195 (86.1401, 51.2254) -> (86.1665, 51.2363)
  line L1196 (86.192, 51.2491) -> (86.2166, 51.2636)
  line L1197 (86.0854, 51.2093) -> (86.113, 51.2164)
  line L1198 (86.2401, 51.2799) -> (86.2623, 51.2978)
  line L1199 (86.0289, 51.2012) -> (86.0573, 51.2042)
  line L1200 (86.0573, 51.2042) -> (86.0854, 51.2093)
  line L1201 (86.1665, 51.2363) -> (86.192, 51.2491)
  line L1202 (86.2166, 51.2636) -> (86.2401, 51.2799)
  line L1203 (86.3993, 51.5716) -> (86.4004, 51.6001)
  line L1204 (86.3751, 51.4603) -> (86.3841, 51.4874)
  line L1205 (86.2623, 51.2978) -> (86.2832, 51.3173)
  line L1206 (86.3368, 51.3839) -> (86.3514, 51.4084)
  line L1207 (86.3963, 51.5432) -> (86.3993, 51.5716)
  line L1208 (86.3206, 51.3604) -> (86.3368, 51.3839)
  line L1209 (86.3642, 51.434) -> (86.3751, 51.4603)
  line L1210 (86.3912, 51.5151) -> (86.3963, 51.5432)
  line L1211 (86.4003, 54.4065) -> (86.3987, 54.436)
  line L1212 (83.5429, 51.2042) -> (83.5713, 51.2012)
  line L1213 (83.4872, 51.2164) -> (83.5148, 51.2093)
  line L1214 (83.2163, 54.5128) -> (83.2092, 54.4851)
  line L1215 (83.4082, 51.2491) -> (83.4337, 51.2363)
  line L1216 (83.2161, 51.4874) -> (83.2251, 51.4603)
  line L1217 (83.2251, 51.4603) -> (83.236, 51.434)
  line L1218 (83.2976, 51.3382) -> (83.317, 51.3173)
  line L1219 (83.5148, 51.2093) -> (83.5429, 51.2042)
  line L1220 (83.2009, 51.5716) -> (83.2039, 51.5432)
  line L1221 (83.2001, 51.6001) -> (83.1998, 51.6001)
  line L1222 (83.3379, 51.2978) -> (83.3601, 51.2799)
  line L1223 (83.1998, 51.6001) -> (83.2009, 51.5716)
  line L1224 (83.2796, 51.3604) -> (83.2976, 51.3382)
  line L1225 (83.2634, 51.3839) -> (83.2796, 51.3604)
  line L1226 (83.209, 51.5151) -> (83.2161, 51.4874)
  line L1227 (83.2092, 54.4851) -> (83.2041, 54.4571)
  line L1228 (83.2001, 54.4001) -> (83.2001, 51.6001)
  line L1229 (83.317, 51.3173) -> (83.3379, 51.2978)
  line L1230 (83.236, 51.434) -> (83.2488, 51.4084)
  line L1231 (83.2039, 51.5432) -> (83.209, 51.5151)
  line L1232 (83.2635, 54.6164) -> (83.249, 54.5918)
  line L1233 (83.2011, 54.4287) -> (83.2001, 54.4001)
  line L1234 (83.4337, 51.2363) -> (83.4601, 51.2254)
  line L1235 (83.2488, 51.4084) -> (83.2634, 51.3839)
  line L1236 (83.2041, 54.4571) -> (83.2011, 54.4287)
  line L1237 (83.3172, 54.683) -> (83.2977, 54.6621)
  line L1238 (83.2798, 54.6398) -> (83.2635, 54.6164)
  line L1239 (83.2253, 54.5399) -> (83.2163, 54.5128)
  line L1240 (83.2977, 54.6621) -> (83.2798, 54.6398)
  line L1241 (83.3603, 54.7203) -> (83.3381, 54.7024)
  line L1242 (83.3838, 54.7366) -> (83.3603, 54.7203)
  line L1243 (83.4602, 54.7749) -> (83.4339, 54.764)
  line L1244 (83.2362, 54.5663) -> (83.2253, 54.5399)
  line L1245 (83.4083, 54.7512) -> (83.3838, 54.7366)
  line L1246 (83.5431, 54.7961) -> (83.515, 54.791)
  line L1247 (83.515, 54.791) -> (83.4873, 54.7839)
  line L1248 (83.4339, 54.764) -> (83.4083, 54.7512)
  line L1249 (83.4873, 54.7839) -> (83.4602, 54.7749)
  line L1250 (83.3381, 54.7024) -> (83.3172, 54.683)
  line L1251 (86.1451, 54.773) -> (86.1171, 54.7827)
  line L1252 (86.0005, 54.8001) -> (86.0001, 54.8001)
  line L1253 (86.0299, 54.799) -> (86.0004, 54.8001)
  line L1254 (86.0594, 54.7957) -> (86.0299, 54.799)
  line L1255 (86.0885, 54.7903) -> (86.0594, 54.7957)
  line L1256 (86.1171, 54.7827) -> (86.0885, 54.7903)
  line L1257 (86.1723, 54.7613) -> (86.1451, 54.773)
  line L1258 (83.6, 54.8001) -> (83.5715, 54.7991)
  line L1259 (83.5715, 54.7991) -> (83.5431, 54.7961)
  line L1260 (86.0001, 54.8001) -> (83.6, 54.8001)
  line L1261 (86.0004, 54.8001) -> (86.0005, 54.8001)
  line L1262 (86.4004, 51.6001) -> (86.4002, 51.6001)
  line L1263 (86.3841, 51.4874) -> (86.3912, 51.5151)
  line L1264 (86.3026, 51.3382) -> (86.3206, 51.3604)
  line L1265 (86.4002, 54.4001) -> (86.4003, 54.4065)
  line L1266 (86.395, 54.4654) -> (86.3891, 54.4944)
  line L1267 (86.3987, 54.436) -> (86.395, 54.4654)
  line L1268 (86.3286, 54.6287) -> (86.3108, 54.6523)
  line L1269 (86.2476, 54.7145) -> (86.2237, 54.732)
  line L1270 (86.2237, 54.732) -> (86.1985, 54.7476)
  line L1271 (86.2702, 54.6954) -> (86.2476, 54.7145)
  line L1272 (86.3446, 54.6038) -> (86.3286, 54.6287)
  line L1273 (86.3588, 54.5777) -> (86.3446, 54.6038)
  line L1274 (86.3709, 54.5507) -> (86.3588, 54.5777)
  line L1275 (86.4002, 51.6001) -> (86.4002, 54.4001)
  line L1276 (86.2832, 51.3173) -> (86.3026, 51.3382)
  line L1277 (86.3891, 54.4944) -> (86.381, 54.5229)
  line L1278 (86.3514, 51.4084) -> (86.3642, 51.434)
  line L1279 (86.381, 54.5229) -> (86.3709, 54.5507)
  line L1280 (86.4002, 74.4001) -> (86.4003, 74.4065)
  line L1281 (83.3381, 74.7024) -> (83.3172, 74.683)
  line L1282 (86.381, 74.5229) -> (86.3709, 74.5507)
  line L1283 (86.395, 74.4654) -> (86.3891, 74.4944)
  line L1284 (83.3838, 74.7366) -> (83.3603, 74.7203)
  line L1285 (83.3603, 74.7203) -> (83.3381, 74.7024)
  line L1286 (86.3987, 74.436) -> (86.395, 74.4654)
  line L1287 (86.4003, 74.4065) -> (86.3987, 74.436)
  line L1288 (83.2001, 74.4001) -> (83.2001, 71.6001)
  line L1289 (86.4004, 71.6001) -> (86.4002, 71.6001)
  line L1290 (83.2001, 71.6001) -> (83.1998, 71.6001)
  line L1291 (83.2011, 74.4287) -> (83.2001, 74.4001)
  line L1292 (83.2634, 71.3839) -> (83.2796, 71.3604)
  line L1293 (83.2039, 71.5432) -> (83.209, 71.5151)
  line L1294 (83.2488, 71.4084) -> (83.2634, 71.3839)
  line L1295 (86.3642, 71.434) -> (86.3751, 71.4603)
  line L1296 (83.2163, 74.5128) -> (83.2092, 74.4851)
  line L1297 (83.1998, 71.6001) -> (83.2009, 71.5716)
  line L1298 (86.4002, 71.6001) -> (86.4002, 74.4001)
  line L1299 (83.2796, 71.3604) -> (83.2976, 71.3382)
  line L1300 (86.2166, 71.2636) -> (86.2401, 71.2799)
  line L1301 (86.0573, 71.2042) -> (86.0854, 71.2093)
  line L1302 (86.3286, 74.6287) -> (86.3108, 74.6523)
  line L1303 (86.0004, 71.2002) -> (86.0289, 71.2012)
  line L1304 (83.4339, 74.764) -> (83.4083, 74.7512)
  line L1305 (86.2623, 71.2978) -> (86.2832, 71.3173)
  line L1306 (83.3172, 74.683) -> (83.2977, 74.6621)
  line L1307 (83.4602, 74.7749) -> (83.4339, 74.764)
  line L1308 (83.5715, 74.7991) -> (83.5431, 74.7961)
  line L1309 (86.3963, 71.5432) -> (86.3993, 71.5716)
  line L1310 (86.3841, 71.4874) -> (86.3912, 71.5151)
  line L1311 (86.2913, 74.6746) -> (86.2702, 74.6954)
  line L1312 (86.3912, 71.5151) -> (86.3963, 71.5432)
  line L1313 (86.1451, 74.773) -> (86.1171, 74.7827)
  line L1314 (83.4873, 74.7839) -> (83.4602, 74.7749)
  line L1315 (86.2237, 74.732) -> (86.1985, 74.7476)
  line L1316 (83.515, 74.791) -> (83.4873, 74.7839)
  line L1317 (86.0001, 74.8001) -> (83.6, 74.8001)
  line L1318 (83.5431, 74.7961) -> (83.515, 74.791)
  line L1319 (86.0005, 74.8001) -> (86.0001, 74.8001)
  line L1320 (86.0299, 74.799) -> (86.0004, 74.8001)
  line L1321 (86.0594, 74.7957) -> (86.0299, 74.799)
  line L1322 (86.0004, 74.8001) -> (86.0005, 74.8001)
  line L1323 (86.3206, 71.3604) -> (86.3368, 71.3839)
  line L1324 (86.3026, 71.3382) -> (86.3206, 71.3604)
  line L1325 (86.2832, 71.3173) -> (86.3026, 71.3382)
  line L1326 (83.6, 74.8001) -> (83.5715, 74.7991)
  line L1327 (86.3891, 74.4944) -> (86.381, 74.5229)
  line L1328 (83.5998, 71.2002) -> (86.0004, 71.2002)
  line L1329 (86.3514, 71.4084) -> (86.3642, 71.434)
  line L1330 (86.0885, 74.7903) -> (86.0594, 74.7957)
  line L1331 (86.3108, 74.6523) -> (86.2913, 74.6746)
  line L1332 (86.1171, 74.7827) -> (86.0885, 74.7903)
  line L1333 (86.1723, 74.7613) -> (86.1451, 74.773)
  line L1334 (86.3993, 71.5716) -> (86.4004, 71.6001)
  line L1335 (86.0289, 71.2012) -> (86.0573, 71.2042)
  line L1336 (83.4872, 71.2164) -> (83.5148, 71.2093)
  line L1337 (86.1985, 74.7476) -> (86.1723, 74.7613)
  line L1338 (86.2476, 74.7145) -> (86.2237, 74.732)
  line L1339 (86.2702, 74.6954) -> (86.2476, 74.7145)
  line L1340 (86.3446, 74.6038) -> (86.3286, 74.6287)
  line L1341 (83.4601, 71.2254) -> (83.4872, 71.2164)
  line L1342 (83.4337, 71.2363) -> (83.4601, 71.2254)
  line L1343 (86.3709, 74.5507) -> (86.3588, 74.5777)
  line L1344 (83.5148, 71.2093) -> (83.5429, 71.2042)
  line L1345 (83.5713, 71.2012) -> (83.5998, 71.2002)
  line L1346 (83.5429, 71.2042) -> (83.5713, 71.2012)
  line L1347 (83.2251, 71.4603) -> (83.236, 71.434)
  line L1348 (83.3836, 71.2636) -> (83.4082, 71.2491)
  line L1349 (83.317, 71.3173) -> (83.3379, 71.2978)
  line L1350 (83.3601, 71.2799) -> (83.3836, 71.2636)
  line L1351 (83.4082, 71.2491) -> (83.4337, 71.2363)
  line L1352 (83.2161, 71.4874) -> (83.2251, 71.4603)
  line L1353 (83.2092, 74.4851) -> (83.2041, 74.4571)
  line L1354 (83.3379, 71.2978) -> (83.3601, 71.2799)
  line L1355 (86.3368, 71.3839) -> (86.3514, 71.4084)
  line L1356 (86.3751, 71.4603) -> (86.3841, 71.4874)
  line L1357 (86.0854, 71.2093) -> (86.113, 71.2164)
  line L1358 (86.113, 71.2164) -> (86.1401, 71.2254)
  line L1359 (86.192, 71.2491) -> (86.2166, 71.2636)
  line L1360 (86.2401, 71.2799) -> (86.2623, 71.2978)
  line L1361 (86.1665, 71.2363) -> (86.192, 71.2491)
  line L1362 (86.1401, 71.2254) -> (86.1665, 71.2363)
  line L1363 (83.2362, 74.5663) -> (83.2253, 74.5399)
  line L1364 (83.249, 74.5918) -> (83.2362, 74.5663)
  line L1365 (83.2798, 74.6398) -> (83.2635, 74.6164)
  line L1366 (83.2253, 74.5399) -> (83.2163, 74.5128)
  line L1367 (83.4083, 74.7512) -> (83.3838, 74.7366)
  line L1368 (83.2977, 74.6621) -> (83.2798, 74.6398)
  line L1369 (83.2635, 74.6164) -> (83.249, 74.5918)
  line L1370 (86.3588, 74.5777) -> (86.3446, 74.6038)
  line L1371 (83.209, 71.5151) -> (83.2161, 71.4874)
  line L1372 (83.236, 71.434) -> (83.2488, 71.4084)
  line L1373 (83.2976, 71.3382) -> (83.317, 71.3173)
  line L1374 (83.2041, 74.4571) -> (83.2011, 74.4287)
  line L1375 (83.2009, 71.5716) -> (83.2039, 71.5432)
  line L1376 (71.2976, 83.3381) -> (71.317, 83.3172)
  line L1377 (71.5429, 83.2041) -> (71.5713, 83.2011)
  line L1378 (74.4284, 83.2009) -> (74.4568, 83.2039)
  line L1379 (71.5999, 83.2001) -> (74.3999, 83.2001)
  line L1380 (71.5149, 83.2092) -> (71.5429, 83.2041)
  line L1381 (71.3379, 83.2977) -> (71.3602, 83.2798)
  line L1382 (71.2634, 83.3838) -> (71.2797, 83.3603)
  line L1383 (71.2488, 83.4083) -> (71.2634, 83.3838)
  line L1384 (71.4337, 83.2362) -> (71.4601, 83.2253)
  line L1385 (71.2251, 83.4602) -> (71.236, 83.4339)
  line L1386 (71.2797, 83.3603) -> (71.2976, 83.3381)
  line L1387 (71.3836, 83.2635) -> (71.4082, 83.249)
  line L1388 (71.2161, 83.4873) -> (71.2251, 83.4602)
  line L1389 (71.3602, 83.2798) -> (71.3836, 83.2635)
  line L1390 (71.317, 83.3172) -> (71.3379, 83.2977)
  line L1391 (71.236, 83.4339) -> (71.2488, 83.4083)
  line L1392 (71.2039, 83.5431) -> (71.209, 83.515)
  line L1393 (71.209, 83.515) -> (71.2161, 83.4873)
  line L1394 (71.2009, 83.5715) -> (71.2039, 83.5431)
  line L1395 (71.2097, 86.0885) -> (71.2043, 86.0594)
  line L1396 (71.1999, 86.0005) -> (71.1999, 86.0001)
  line L1397 (71.2043, 86.0594) -> (71.201, 86.0299)
  line L1398 (71.2173, 86.1171) -> (71.2097, 86.0885)
  line L1399 (71.1999, 86.0001) -> (71.1999, 83.6)
  line L1400 (71.1999, 83.6) -> (71.2009, 83.5715)
  line L1401 (71.1999, 86.0004) -> (71.1999, 86.0005)
  line L1402 (71.201, 86.0299) -> (71.1999, 86.0004)
  line L1403 (71.2855, 86.2476) -> (71.268, 86.2237)
  line L1404 (71.5056, 86.3891) -> (71.4771, 86.381)
  line L1405 (71.3254, 86.2913) -> (71.3046, 86.2702)
  line L1406 (71.4223, 86.3588) -> (71.3962, 86.3446)
  line L1407 (71.227, 86.1451) -> (71.2173, 86.1171)
  line L1408 (71.2387, 86.1723) -> (71.227, 86.1451)
  line L1409 (71.268, 86.2237) -> (71.2524, 86.1985)
  line L1410 (71.2524, 86.1985) -> (71.2387, 86.1723)
  line L1411 (71.3962, 86.3446) -> (71.3713, 86.3286)
  line L1412 (71.3713, 86.3286) -> (71.3477, 86.3108)
  line L1413 (71.3477, 86.3108) -> (71.3254, 86.2913)
  line L1414 (71.4771, 86.381) -> (71.4493, 86.3709)
  line L1415 (71.3046, 86.2702) -> (71.2855, 86.2476)
  line L1416 (71.4493, 86.3709) -> (71.4223, 86.3588)
  line L1417 (74.4849, 86.3912) -> (74.4568, 86.3963)
  line L1418 (71.5935, 86.4003) -> (71.564, 86.3987)
  line L1419 (71.5346, 86.395) -> (71.5056, 86.3891)
  line L1420 (71.564, 86.3987) -> (71.5346, 86.395)
  line L1421 (74.3999, 83.1998) -> (74.4284, 83.2009)
  line L1422 (74.4568, 86.3963) -> (74.4284, 86.3993)
  line L1423 (74.5397, 83.2251) -> (74.566, 83.236)
  line L1424 (74.5916, 83.2488) -> (74.6161, 83.2634)
  line L1425 (71.5713, 83.2011) -> (71.5999, 83.2001)
  line L1426 (71.4601, 83.2253) -> (71.4872, 83.2163)
  line L1427 (74.3999, 83.2001) -> (74.3999, 83.1998)
  line L1428 (71.4082, 83.249) -> (71.4337, 83.2362)
  line L1429 (74.3999, 86.4004) -> (74.3999, 86.4002)
  line L1430 (71.5999, 86.4002) -> (71.5935, 86.4003)
  line L1431 (74.4284, 86.3993) -> (74.3999, 86.4004)
  line L1432 (74.6161, 86.3368) -> (74.5916, 86.3514)
  line L1433 (74.5397, 86.3751) -> (74.5126, 86.3841)
  line L1434 (74.566, 86.3642) -> (74.5397, 86.3751)
  line L1435 (74.3999, 86.4002) -> (71.5999, 86.4002)
  line L1436 (74.5916, 86.3514) -> (74.566, 86.3642)
  line L1437 (74.5126, 86.3841) -> (74.4849, 86.3912)
  line L1438 (74.4849, 83.209) -> (74.5126, 83.2161)
  line L1439 (74.6827, 83.317) -> (74.7022, 83.3379)
  line L1440 (74.7022, 83.3379) -> (74.7201, 83.3601)
  line L1441 (74.566, 83.236) -> (74.5916, 83.2488)
  line L1442 (74.4568, 83.2039) -> (74.4849, 83.209)
  line L1443 (71.4872, 83.2163) -> (71.5149, 83.2092)
  line L1444 (74.6396, 83.2796) -> (74.6618, 83.2976)
  line L1445 (74.6161, 83.2634) -> (74.6396, 83.2796)
  line L1446 (74.5126, 83.2161) -> (74.5397, 83.2251)
  line L1447 (74.6618, 83.2976) -> (74.6827, 83.317)
  line L1448 (74.7364, 86.2166) -> (74.7201, 86.2401)
  line L1449 (74.7907, 86.0854) -> (74.7836, 86.113)
  line L1450 (74.7746, 86.1401) -> (74.7637, 86.1665)
  line L1451 (74.6827, 86.2832) -> (74.6618, 86.3026)
  line L1452 (74.7637, 86.1665) -> (74.7509, 86.192)
  line L1453 (74.7201, 86.2401) -> (74.7022, 86.2623)
  line L1454 (74.6396, 86.3206) -> (74.6161, 86.3368)
  line L1455 (74.7836, 86.113) -> (74.7746, 86.1401)
  line L1456 (74.7509, 86.192) -> (74.7364, 86.2166)
  line L1457 (74.7022, 86.2623) -> (74.6827, 86.2832)
  line L1458 (74.6618, 86.3026) -> (74.6396, 86.3206)
  line L1459 (74.7958, 86.0573) -> (74.7907, 86.0854)
  line L1460 (74.7998, 86.0004) -> (74.7988, 86.0289)
  line L1461 (74.7988, 86.0289) -> (74.7958, 86.0573)
  line L1462 (74.7509, 83.4082) -> (74.7637, 83.4337)
  line L1463 (74.7746, 83.4601) -> (74.7836, 83.4872)
  line L1464 (74.7988, 83.5713) -> (74.7998, 83.5998)
  line L1465 (74.7364, 83.3836) -> (74.7509, 83.4082)
  line L1466 (74.7998, 83.5998) -> (74.7998, 86.0004)
  line L1467 (74.7201, 83.3601) -> (74.7364, 83.3836)
  line L1468 (74.7836, 83.4872) -> (74.7907, 83.5148)
  line L1469 (74.7907, 83.5148) -> (74.7958, 83.5429)
  line L1470 (74.7958, 83.5429) -> (74.7988, 83.5713)
  line L1471 (74.7637, 83.4337) -> (74.7746, 83.4601)
  line L1472 (51.5935, 86.4003) -> (51.564, 86.3987)
  line L1473 (51.2855, 86.2476) -> (51.268, 86.2237)
  line L1474 (54.3999, 86.4002) -> (51.5999, 86.4002)
  line L1475 (51.5999, 86.4002) -> (51.5935, 86.4003)
  line L1476 (54.3999, 86.4004) -> (54.3999, 86.4002)
  line L1477 (54.5916, 86.3514) -> (54.566, 86.3642)
  line L1478 (54.4849, 86.3912) -> (54.4568, 86.3963)
  line L1479 (54.5397, 86.3751) -> (54.5126, 86.3841)
  line L1480 (54.7998, 86.0004) -> (54.7988, 86.0289)
  line L1481 (54.7509, 86.192) -> (54.7364, 86.2166)
  line L1482 (54.566, 86.3642) -> (54.5397, 86.3751)
  line L1483 (54.7907, 86.0854) -> (54.7836, 86.113)
  line L1484 (54.4284, 86.3993) -> (54.3999, 86.4004)
  line L1485 (51.2039, 83.5431) -> (51.209, 83.515)
  line L1486 (54.7637, 86.1665) -> (54.7509, 86.192)
  line L1487 (54.7958, 86.0573) -> (54.7907, 86.0854)
  line L1488 (51.3046, 86.2702) -> (51.2855, 86.2476)
  line L1489 (54.7201, 86.2401) -> (54.7022, 86.2623)
  line L1490 (51.1999, 86.0001) -> (51.1999, 83.6)
  line L1491 (54.6396, 86.3206) -> (54.6161, 86.3368)
  line L1492 (54.5126, 83.2161) -> (54.5397, 83.2251)
  line L1493 (54.7746, 86.1401) -> (54.7637, 86.1665)
  line L1494 (51.2634, 83.3838) -> (51.2797, 83.3603)
  line L1495 (54.7988, 86.0289) -> (54.7958, 86.0573)
  line L1496 (51.2488, 83.4083) -> (51.2634, 83.3838)
  line L1497 (54.7364, 86.2166) -> (54.7201, 86.2401)
  line L1498 (54.5126, 86.3841) -> (54.4849, 86.3912)
  line L1499 (54.6161, 86.3368) -> (54.5916, 86.3514)
  line L1500 (51.2524, 86.1985) -> (51.2387, 86.1723)
  line L1501 (54.7836, 86.113) -> (54.7746, 86.1401)
  line L1502 (54.5397, 83.2251) -> (54.566, 83.236)
  line L1503 (54.5916, 83.2488) -> (54.6161, 83.2634)
  line L1504 (51.4601, 83.2253) -> (51.4872, 83.2163)
  line L1505 (54.6618, 83.2976) -> (54.6827, 83.317)
  line L1506 (51.3477, 86.3108) -> (51.3254, 86.2913)
  line L1507 (51.5056, 86.3891) -> (51.4771, 86.381)
  line L1508 (54.6161, 83.2634) -> (54.6396, 83.2796)
  line L1509 (51.3254, 86.2913) -> (51.3046, 86.2702)
  line L1510 (51.2043, 86.0594) -> (51.201, 86.0299)
  line L1511 (51.2251, 83.4602) -> (51.236, 83.4339)
  line L1512 (51.4872, 83.2163) -> (51.5149, 83.2092)
  line L1513 (51.1999, 83.6) -> (51.2009, 83.5715)
  line L1514 (51.3602, 83.2798) -> (51.3836, 83.2635)
  line L1515 (54.7509, 83.4082) -> (54.7637, 83.4337)
  line L1516 (51.4082, 83.249) -> (51.4337, 83.2362)
  line L1517 (54.6827, 83.317) -> (54.7022, 83.3379)
  line L1518 (51.268, 86.2237) -> (51.2524, 86.1985)
  line L1519 (51.4223, 86.3588) -> (51.3962, 86.3446)
  line L1520 (54.7022, 83.3379) -> (54.7201, 83.3601)
  line L1521 (51.1999, 86.0004) -> (51.1999, 86.0005)
  line L1522 (51.2009, 83.5715) -> (51.2039, 83.5431)
  line L1523 (54.4568, 83.2039) -> (54.4849, 83.209)
  line L1524 (51.5999, 83.2001) -> (54.3999, 83.2001)
  line L1525 (51.4337, 83.2362) -> (51.4601, 83.2253)
  line L1526 (54.4849, 83.209) -> (54.5126, 83.2161)
  line L1527 (54.6396, 83.2796) -> (54.6618, 83.2976)
  line L1528 (51.5713, 83.2011) -> (51.5999, 83.2001)
  line L1529 (54.3999, 83.2001) -> (54.3999, 83.1998)
  line L1530 (51.1999, 86.0005) -> (51.1999, 86.0001)
  line L1531 (54.4284, 83.2009) -> (54.4568, 83.2039)
  line L1532 (51.317, 83.3172) -> (51.3379, 83.2977)
  line L1533 (51.2797, 83.3603) -> (51.2976, 83.3381)
  line L1534 (51.2976, 83.3381) -> (51.317, 83.3172)
  line L1535 (51.2173, 86.1171) -> (51.2097, 86.0885)
  line L1536 (51.564, 86.3987) -> (51.5346, 86.395)
  line L1537 (51.2161, 83.4873) -> (51.2251, 83.4602)
  line L1538 (51.3836, 83.2635) -> (51.4082, 83.249)
  line L1539 (51.2387, 86.1723) -> (51.227, 86.1451)
  line L1540 (54.6827, 86.2832) -> (54.6618, 86.3026)
  line L1541 (54.7836, 83.4872) -> (54.7907, 83.5148)
  line L1542 (51.209, 83.515) -> (51.2161, 83.4873)
  line L1543 (54.7637, 83.4337) -> (54.7746, 83.4601)
  line L1544 (51.4493, 86.3709) -> (51.4223, 86.3588)
  line L1545 (51.5149, 83.2092) -> (51.5429, 83.2041)
  line L1546 (51.201, 86.0299) -> (51.1999, 86.0004)
  line L1547 (54.7201, 83.3601) -> (54.7364, 83.3836)
  line L1548 (51.236, 83.4339) -> (51.2488, 83.4083)
  line L1549 (54.7958, 83.5429) -> (54.7988, 83.5713)
  line L1550 (54.7746, 83.4601) -> (54.7836, 83.4872)
  line L1551 (54.7364, 83.3836) -> (54.7509, 83.4082)
  line L1552 (54.7998, 83.5998) -> (54.7998, 86.0004)
  line L1553 (51.3379, 83.2977) -> (51.3602, 83.2798)
  line L1554 (51.2097, 86.0885) -> (51.2043, 86.0594)
  line L1555 (51.5429, 83.2041) -> (51.5713, 83.2011)
  line L1556 (54.7907, 83.5148) -> (54.7958, 83.5429)
  line L1557 (54.7988, 83.5713) -> (54.7998, 83.5998)
  line L1558 (51.3962, 86.3446) -> (51.3713, 86.3286)
  line L1559 (54.566, 83.236) -> (54.5916, 83.2488)
  line L1560 (51.227, 86.1451) -> (51.2173, 86.1171)
  line L1561 (51.5346, 86.395) -> (51.5056, 86.3891)
  line L1562 (54.3999, 83.1998) -> (54.4284, 83.2009)
  line L1563 (51.4771, 86.381) -> (51.4493, 86.3709)
  line L1564 (54.7022, 86.2623) -> (54.6827, 86.2832)
  line L1565 (51.3713, 86.3286) -> (51.3477, 86.3108)
  line L1566 (54.6618, 86.3026) -> (54.6396, 86.3206)
  line L1567 (54.4568, 86.3963) -> (54.4284, 86.3993)
  line L1568 (34.7988, 86.0289) -> (34.7958, 86.0573)
  line L1569 (31.236, 83.4339) -> (31.2488, 83.4083)
  line L1570 (34.7998, 86.0004) -> (34.7988, 86.0289)
  line L1571 (34.4849, 86.3912) -> (34.4568, 86.3963)
  line L1572 (34.6396, 86.3206) -> (34.6161, 86.3368)
  line L1573 (34.3999, 86.4002) -> (31.5999, 86.4002)
  line L1574 (34.4284, 86.3993) -> (34.3999, 86.4004)
  line L1575 (31.2009, 83.5715) -> (31.2039, 83.5431)
  line L1576 (34.6161, 83.2634) -> (34.6396, 83.2796)
  line L1577 (31.4771, 86.381) -> (31.4493, 86.3709)
  line L1578 (34.6618, 86.3026) -> (34.6396, 86.3206)
  line L1579 (34.5397, 86.3751) -> (34.5126, 86.3841)
  line L1580 (34.6161, 86.3368) -> (34.5916, 86.3514)
  line L1581 (31.2387, 86.1723) -> (31.227, 86.1451)
  line L1582 (31.201, 86.0299) -> (31.1999, 86.0004)
  line L1583 (31.1999, 86.0004) -> (31.1999, 86.0005)
  line L1584 (34.7201, 86.2401) -> (34.7022, 86.2623)
  line L1585 (31.5935, 86.4003) -> (31.564, 86.3987)
  line L1586 (31.5056, 86.3891) -> (31.4771, 86.381)
  line L1587 (31.3477, 86.3108) -> (31.3254, 86.2913)
  line L1588 (31.5999, 86.4002) -> (31.5935, 86.4003)
  line L1589 (34.7509, 86.192) -> (34.7364, 86.2166)
  line L1590 (34.4568, 86.3963) -> (34.4284, 86.3993)
  line L1591 (34.3999, 86.4004) -> (34.3999, 86.4002)
  line L1592 (31.227, 86.1451) -> (31.2173, 86.1171)
  line L1593 (31.564, 86.3987) -> (31.5346, 86.395)
  line L1594 (34.5916, 86.3514) -> (34.566, 86.3642)
  line L1595 (31.2173, 86.1171) -> (31.2097, 86.0885)
  line L1596 (31.2976, 83.3381) -> (31.317, 83.3172)
  line L1597 (34.7364, 83.3836) -> (34.7509, 83.4082)
  line L1598 (31.1999, 83.6) -> (31.2009, 83.5715)
  line L1599 (34.7746, 86.1401) -> (34.7637, 86.1665)
  line L1600 (31.3046, 86.2702) -> (31.2855, 86.2476)
  line L1601 (34.7998, 83.5998) -> (34.7998, 86.0004)
  line L1602 (34.566, 83.236) -> (34.5916, 83.2488)
  line L1603 (34.7637, 83.4337) -> (34.7746, 83.4601)
  line L1604 (34.5397, 83.2251) -> (34.566, 83.236)
  line L1605 (31.3254, 86.2913) -> (31.3046, 86.2702)
  line L1606 (34.7907, 86.0854) -> (34.7836, 86.113)
  line L1607 (34.7364, 86.2166) -> (34.7201, 86.2401)
  line L1608 (31.4493, 86.3709) -> (31.4223, 86.3588)
  line L1609 (31.3713, 86.3286) -> (31.3477, 86.3108)
  line L1610 (31.2043, 86.0594) -> (31.201, 86.0299)
  line L1611 (34.7637, 86.1665) -> (34.7509, 86.192)
  line L1612 (31.209, 83.515) -> (31.2161, 83.4873)
  line L1613 (31.3962, 86.3446) -> (31.3713, 86.3286)
  line L1614 (34.5126, 86.3841) -> (34.4849, 86.3912)
  line L1615 (34.6827, 86.2832) -> (34.6618, 86.3026)
  line L1616 (34.7958, 83.5429) -> (34.7988, 83.5713)
  line L1617 (31.3602, 83.2798) -> (31.3836, 83.2635)
  line L1618 (34.7958, 86.0573) -> (34.7907, 86.0854)
  line L1619 (31.268, 86.2237) -> (31.2524, 86.1985)
  line L1620 (31.2797, 83.3603) -> (31.2976, 83.3381)
  line L1621 (34.566, 86.3642) -> (34.5397, 86.3751)
  line L1622 (31.2097, 86.0885) -> (31.2043, 86.0594)
  line L1623 (31.5346, 86.395) -> (31.5056, 86.3891)
  line L1624 (31.2524, 86.1985) -> (31.2387, 86.1723)
  line L1625 (34.7836, 86.113) -> (34.7746, 86.1401)
  line L1626 (31.2039, 83.5431) -> (31.209, 83.515)
  line L1627 (31.1999, 86.0001) -> (31.1999, 83.6)
  line L1628 (31.5999, 83.2001) -> (34.3999, 83.2001)
  line L1629 (31.2634, 83.3838) -> (31.2797, 83.3603)
  line L1630 (34.4849, 83.209) -> (34.5126, 83.2161)
  line L1631 (31.3379, 83.2977) -> (31.3602, 83.2798)